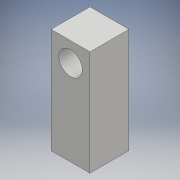
# Autodesk Inventor part: Raket_Arme
Saved by Autodesk Inventor 2018 (Build 220112000, 112)
## iProperties
Created: 2017-08-14
Part Number: Raket_Arme
Material: Generic
Document SubType Name: Modeling
Designer: andre
Density: 1 g/cm^3
Appearance: Default
Author: andre
## iProperties of the stored document Raket_Arme_3DPrint.ipt
Created: 2017-08-14
Part Number: Raket_Arme_3DPrint
Material: Generic
Document SubType Name: Modeling
Designer: andre
Density: 1 g/cm^3
Appearance: Default
Author: andre
Autodesk Inventor part; units mm, degrees
ref_plane "YZ Plane" through (0, 0, 0) normal (1, 0, 0) x (0, 1, 0)
ref_plane "XZ Plane" through (0, 0, 0) normal (0, 1, 0) x (-1, 0, 0)
ref_plane "XY Plane" through (0, 0, 0) normal (0, 0, 1) x (1, 0, 0)
sketch "Sketch1" plane through (0, 0, 0) normal (0, 1, 0) x (-1, 0, 0)
  line L0 (0, 0) -> (10, 0)
  line L1 (10, 0) -> (10, -27)
  line L2 (10, -27) -> (0, -27)
  line L3 (0, -27) -> (0, 0)
  dimension "d0" = 10
  dimension "d1" = 27
  constraints: 8 end point, 2 parallel, 1 horizontal, 1 perpendicular
  measures "d0" distance of L1.end L2.end
  measures "d1" distance of L0.end L1.end
extrude "Extrusion1" add sketch "Sketch1" along normal blind 10
sketch "Sketch2" plane through (0, 10, 0) normal (0, 1, 0) x (1, 0, 0)
  line L0 (-10, 27) -> (-10, 0) projected
  line L1 (-10, 0) -> (-10, 5)
  circle A0 centre (-5, 5) radius 3
  point P0 (0, 0)
  dimension "d4" = 5
  dimension "d5" = 6
  constraints: 2 end point, 1 centre point, 1 point on line
  measures "d4" distance of L0.end L1.end
  measures "d5" diameter of A0
extrude "Extrusion2" cut sketch "Sketch2" against normal blind 10
sketch "Sketch3" plane through (0, 0, -27) normal (0, 0, -1) x (-1, 0, 0)
  line L0 (0, 10) -> (10, 10) projected
  line L1 (0, 10) -> (5, 10)
  line L2 (5, 10) -> (5, 5)
  circle A0 centre (5, 5) radius 1.95
  point P0 (0, 0)
  dimension "d8" = 5
  dimension "d9" = 5
  dimension "d10" = 3.9
  constraints: 4 end point, 1 centre point, 1 coincident, 1 midpoint, 1 perpendicular
  measures "d8" distance of L0.start L1.end
  measures "d9" distance of L1.end L2.end
  measures "d10" diameter of A0
extrude "Extrusion3" cut sketch "Sketch3" against normal blind 15
body "Solid1"
